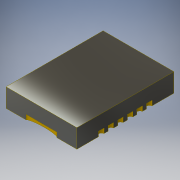
# Autodesk Inventor part: MC_DK1042
Saved by Autodesk Inventor 2016 (Build 200138000, 138)
## iProperties
Created: 2016-08-30
Part Number: MC_DK1042
Material: Generic
Document SubType Name: Modeling
Designer: jfixelle
Density: 1 g/cm^3
Appearance: Silver
Author: jfixelle
Autodesk Inventor part; units mm, degrees
ref_plane "YZ Plane" through (0, 0, 0) normal (1, 0, 0) x (0, 1, 0)
ref_plane "XZ Plane" through (0, 0, 0) normal (0, 1, 0) x (-1, 0, 0)
ref_plane "XY Plane" through (0, 0, 0) normal (0, 0, 1) x (1, 0, 0)
sketch "Sketch1" plane through (0, 0, 0) normal (0, 1, 0) x (-1, 0, 0)
  line L0 (7.415, 10.16) -> (-7.415, 10.16)
  line L1 (-7.415, 10.16) -> (-7.415, -10.16)
  line L2 (-7.415, -10.16) -> (7.415, -10.16)
  line L3 (7.415, -10.16) -> (7.415, 10.16)
  point P0 (0, 0)
  dimension "d0" = 20.32
  dimension "d1" = 10.16
  dimension "d2" = 14.83
  dimension "d3" = 7.415
  constraints: 8 end point, 2 parallel, 1 horizontal, 1 perpendicular
  measures "d0" distance of L2.end L0.start
  measures "d1" distance from line of L2 point (0, 0)
  measures "d2" distance between parallel lines of L1 L3
  measures "d3" distance from line of L3 point (0, 0)
extrude "Extrusion1" add sketch "Sketch1" along normal blind 3.91
sketch "Sketch2" plane through (0, 0, 0) normal (0, 1, 0) x (-1, 0, 0)
  line L0 (6.465, -5.76) -> (7.465, -5.76)
  line L1 (7.465, -5.76) -> (7.465, -4.24)
  line L2 (7.465, -4.24) -> (6.465, -4.24)
  line L3 (6.465, -4.24) -> (6.465, -5.76)
  line L4 (7.415, -10.16) -> (7.415, 10.16) projected
  line L5 (-7.415, -10.16) -> (7.415, -10.16) projected
  circle A0 centre (7.465, -5) radius 0.5724
  point P0 (0, 0)
  dimension "d6" = 1
  dimension "d7" = 1.52
  dimension "d8" = 0.05
  dimension "d9" = 4.4
  constraints: 8 end point, 2 parallel, 1 centre point, 1 horizontal, 1 midpoint, 1 perpendicular
  measures "d6" distance of L1.end L2.end
  measures "d7" distance of L0.end L1.end
  measures "d8" distance between parallel lines of L4 L1
  measures "d9" distance between parallel lines of L5 L0
extrude "Extrusion2" cut sketch "Sketch2" along normal blind 1 contours A0 L4 | L4 A0 L1 | L1 A0
pattern_linear "Rectangular Pattern1" count 6 spacing 2.01 along (0, 0, 1) of "Extrusion2"
mirror "Mirror1" about plane through (0, 0, 0) normal (1, 0, 0) of "Extrusion2", "Rectangular Pattern1"
sketch "Sketch3" plane through (0, 0, 0) normal (0, -1, 0) x (1, 0, 0)
  line L0 (3.695, -10.21) -> (-3.695, -10.21)
  line L1 (-3.695, -10.21) -> (-3.695, -9.21)
  line L2 (-3.695, -9.21) -> (3.695, -9.21)
  line L3 (3.695, -9.21) -> (3.695, -10.21)
  line L4 (7.415, -10.16) -> (-7.415, -10.16) projected
  ellipse E0 centre (0, -10.21) end of major axis (-3.2399, -10.21) minor radius 0.6001
  point P0 (0, 0)
  dimension "d15" = 0.05
  dimension "d16" = 7.39
  dimension "d17" = 3.695
  dimension "d18" = 1
  constraints: 8 end point, 2 parallel, 1 horizontal, 1 midpoint, 1 perpendicular, 2 other
  measures "d15" distance between parallel lines of L4 L0
  measures "d16" distance of L0.start L0.end
  measures "d17" distance from line of point (0, 0) L3
  measures "d18" distance of L0.end L1.end
extrude "Extrusion3" cut sketch "Sketch3" against normal blind 1 contours E0 L4 L0 | L0 E0 | E0 L4
mirror "Mirror2" about plane through (0, 0, 0) normal (0, 0, 1) of "Extrusion3"
body "Solid1"
